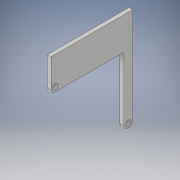
# Autodesk Inventor part: Ventilador bobina - suport
Saved by Autodesk Inventor 2019 (Build 230136000, 136)
## iProperties
Created: 2018-09-18
Part Number: Ventilador bobina - suport
Material: Genérico
Document SubType Name: Modeling
Designer: Albert Garangou Culebras
Density: 1 g/cm^3
Appearance: Valor por defecto
Author: Albert Garangou Culebras
Autodesk Inventor part; units mm, degrees
ref_plane "YZ Plane" through (0, 0, 0) normal (1, 0, 0) x (0, 1, 0)
ref_plane "XZ Plane" through (0, 0, 0) normal (0, 1, 0) x (-1, 0, 0)
ref_plane "XY Plane" through (0, 0, 0) normal (0, 0, 1) x (1, 0, 0)
sketch "Boceto1" plane through (0, 0, 0) normal (1, 0, 0) x (0, 1, 0)
  line L0 (0, 0) -> (0, -3)
  line L1 (0, 0) -> (0, 2.8622)
  line L2 (0, 2.8622) -> (44, 2.8622)
  line L3 (50, -3) -> (0, -3)
  line L4 (50, 0) -> (50, 50)
  line L5 (50, 50) -> (44, 50)
  line L6 (44, 50) -> (44, 2.8622)
  line L7 (50, 0) -> (50, -3)
  circle A0 centre (47, 47.25) radius 1.75
  circle A1 centre (2.75, 0) radius 1.75
  constraints: 17 end point, 4 vertical, 2 centre point, 2 perpendicular, 1 horizontal
sketch "Boceto2" plane through (0, 0, 0) normal (1, 0, 0) x (0, 1, 0)
  line L0 (50, 50) -> (65, 50)
  line L1 (65, 50) -> (65, -3)
  line L2 (65, -3) -> (50, -3)
  line L3 (50, 50) -> (50, -3)
  point P0 (0, 0)
  dimension "d9" = 15
  dimension "d10" = 53
  constraints: 8 end point, 2 perpendicular, 1 horizontal, 1 vertical
  measures "d9" distance of L0.start L0.end
  measures "d10" distance of L0.end L1.end
extrude "Extrusión1" add sketch "Boceto1" along normal blind 2.5
extrude "Extrusión2" add sketch "Boceto2" along normal blind 2.5
fillet "Empalme1" radius 2.9311 2 edges at (1.25, 0, 2.8622) (1.25, 0, -3)
fillet "Empalme2" radius 2.5 1 edges at (1.25, 44, 50)
